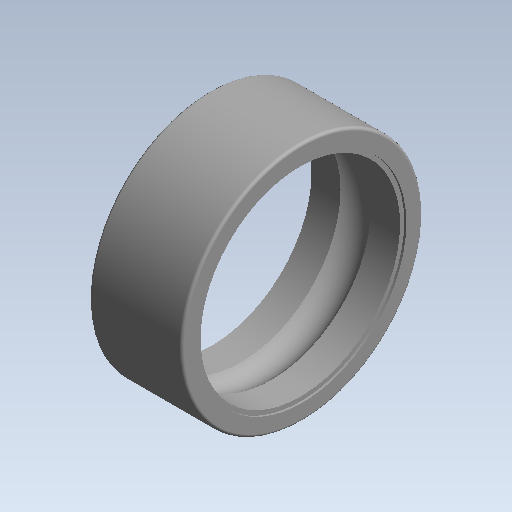
# Autodesk Inventor part: W686ZZ Outer ring
Saved by Autodesk Inventor 2021.3 (Build 253353010, 353A)
## iProperties
Part Number: W686ZZ Outer ring
Material: 一般
Catalog Web Link: www.cadenas.de
Description: Six types or-Metric system sizes
Vendor: NTN
Document SubType Name: Modeling
Designer: partserver
Manufacturer: NTN
Mass: 0.190628 g
Surface Area: 4.63679 cm^2
Volume: 0.190628 cm^3
Density: 1 g/cm^3
Appearance: PSOLRGB-192-192-192
Category: PARTsolutions
Company: NTN
PSOL_IDENT_0: {$CADENAS_DATA\23d-libs\ntn\ball_roller_bearings\miniature_extra_small_bb\metric_system_sizes\mss_or
PSOL_IDENT_1: .prj},183 {VTYP=3D},{NB=W686ZZ Outer ring},{LINA=W686ZZ Outer ring},{NN=Six types or},{DATE=23.10.20
PSOL_IDENT_2: 20 01:13:35},{GEOMDATE=06.03.2020 10:07:12},{VERSION=},{LINEID=12860},{WBVAR=},{WBNUMERIC=}  {NB=W68
PSOL_IDENT_3: 6ZZ Outer ring},{LINA=W686ZZ Outer ring},{KT=DUMMY},{IDNR=},{SD=6.0},{D=13},{B=3.5},{R=0.15},{ORDER=
PSOL_IDENT_4: W686ZZ},{CR=1 080},{COR=440},{CRF=110},{CORF=45},{LSG=39 000},{LSO=46 000},{MASS=1.90},{D1=15.0},{D2=
PSOL_IDENT_5: 15.2},{C1=1.0},{C2=1.1},{ORDER1=686},{WSS=W686ZZ},{WDS=ZZ},{UTWF=FL686},{FORSS=FLW686Z},{FORDS=ZZ},{
PSOL_IDENT_6: DA1=7},{DA2=7,2},{DA=11,8},{RAS=0,15},{MASS1=2.20},{B1=5.0},{VERS=3},{X=3.5},{N=8},{O=29.83},{RB=1.0
PSOL_IDENT_7: 36}
NB: W686ZZ Outer ring
NN: Six types or
NT: Metric system sizes
NBSYN: $ORDER. Outer ring
LINA: W686ZZ Outer ring
CATALOG: NTN Corporation
SD: 6
D: 13
B: 3.5
R: 0.15
CR: 1 080
COR: 440
CRF: 110
CORF: 45
LSG: 39 000
LSO: 46 000
MASS: 1.9
D1: 15
D2: 15.2
C1: 1
C2: 1.1
ORDER1: 686
WSS: W686ZZ
WDS: ZZ
UTWF: FL686
FORSS: FLW686Z
FORDS: ZZ
DA1: 7
DA2: 7,2
DA: 11,8
RAS: 0,15
MASS1: 2.2
B1: 5
VERS: 3
SUPPLIER: NTN
ARTICLENO: W686ZZ Outer ring
BOMINFO: W686ZZ Outer ring
CREATOR: CADENAS GmbH
Title: W686ZZ Outer ring
Author: Cadenas PARTsolutions
Comments: Metric system sizes
Autodesk Inventor part; units mm, degrees
sketch "Sketch_3" plane through (0, 0, 0) normal (0, 0, 1) x (1, 0, 0)
  line L0 (5, 0) -> (0, 0)
  line L1 (0, 5.604) -> (0.1125, 5.604)
  line L2 (0.1125, 5.604) -> (0.1125, 5.38)
  line L3 (0.1125, 5.38) -> (1.6776, 5.38)
  arc A0 (3.3224, 5.38) -> (1.6776, 5.38) centre (2.5, 4.75) ccw
  line L4 (3.3224, 5.38) -> (4.8875, 5.38)
  line L5 (4.8875, 5.38) -> (4.8875, 5.604)
  line L6 (4.8875, 5.604) -> (5, 5.604)
  line L7 (5, 5.604) -> (5, 6.35)
  arc A1 (5, 6.35) -> (4.85, 6.5) centre (4.85, 6.35) ccw
  line L8 (4.85, 6.5) -> (0.15, 6.5)
  arc A2 (0.15, 6.5) -> (0, 6.35) centre (0.15, 6.35) ccw
  line L9 (0, 6.35) -> (0, 5.604)
  constraints: 20 end point, 6 point on circle, 3 centre point
revolve "Revolution1" add sketch "Sketch_3" angle 360 about axis through (5, 0, 0) along (1, 0, 0)
ref_plane "mss_or_XY" through (0, 0, 0) normal (1, 0, 0) x (0, 0, -1)
ref_plane "mss_or_YZ" through (0, 0, 0) normal (0, 0, -1) x (0, 1, 0)
ref_plane "mss_or_ZX" through (0, 0, 0) normal (0, 1, 0) x (1, 0, 0)
ref_plane "mss_or11_XY" through (5, 0, 0) normal (1, 0, 0) x (0, 0, -1)
ref_plane "mss_or11_YZ" through (5, 0, 0) normal (0, 0, -1) x (0, 1, 0)
ref_plane "mss_or11_ZX" through (5, 0, 0) normal (0, 1, 0) x (1, 0, 0)
ref_plane "mss_or2_1_XY" through (1.75, 4.75, 0) normal (1, 0, 0) x (0, 0, -1)
ref_plane "mss_or2_1_YZ" through (1.75, 4.75, 0) normal (0, 0, -1) x (0, 1, 0)
ref_plane "mss_or2_1_ZX" through (1.75, 4.75, 0) normal (0, 1, 0) x (1, 0, 0)
ref_plane "mss_or2_2_XY" through (1.75, 3.3588, 3.3588) normal (1, 0, 0) x (0, 0, -1)
ref_plane "mss_or2_2_YZ" through (1.75, 3.3588, 3.3588) normal (0, 0, -1) x (0, 1, 0)
ref_plane "mss_or2_2_ZX" through (1.75, 3.3588, 3.3588) normal (0, 1, 0) x (1, 0, 0)
ref_plane "mss_or2_3_XY" through (1.75, 0, 4.75) normal (1, 0, 0) x (0, 0, -1)
ref_plane "mss_or2_3_YZ" through (1.75, 0, 4.75) normal (0, 0, -1) x (0, 1, 0)
ref_plane "mss_or2_3_ZX" through (1.75, 0, 4.75) normal (0, 1, 0) x (1, 0, 0)
ref_plane "mss_or2_4_XY" through (1.75, -3.3588, 3.3588) normal (1, 0, 0) x (0, 0, -1)
ref_plane "mss_or2_4_YZ" through (1.75, -3.3588, 3.3588) normal (0, 0, -1) x (0, 1, 0)
ref_plane "mss_or2_4_ZX" through (1.75, -3.3588, 3.3588) normal (0, 1, 0) x (1, 0, 0)
ref_plane "mss_or2_5_XY" through (1.75, -4.75, 0) normal (1, 0, 0) x (0, 0, -1)
ref_plane "mss_or2_5_YZ" through (1.75, -4.75, 0) normal (0, 0, -1) x (0, 1, 0)
ref_plane "mss_or2_5_ZX" through (1.75, -4.75, 0) normal (0, 1, 0) x (1, 0, 0)
ref_plane "mss_or2_6_XY" through (1.75, -3.3588, -3.3588) normal (1, 0, 0) x (0, 0, -1)
ref_plane "mss_or2_6_YZ" through (1.75, -3.3588, -3.3588) normal (0, 0, -1) x (0, 1, 0)
ref_plane "mss_or2_6_ZX" through (1.75, -3.3588, -3.3588) normal (0, 1, 0) x (1, 0, 0)
ref_plane "mss_or2_7_XY" through (1.75, 0, -4.75) normal (1, 0, 0) x (0, 0, -1)
ref_plane "mss_or2_7_YZ" through (1.75, 0, -4.75) normal (0, 0, -1) x (0, 1, 0)
ref_plane "mss_or2_7_ZX" through (1.75, 0, -4.75) normal (0, 1, 0) x (1, 0, 0)
ref_plane "mss_or2_8_XY" through (1.75, 3.3588, -3.3588) normal (1, 0, 0) x (0, 0, -1)
ref_plane "mss_or2_8_YZ" through (1.75, 3.3588, -3.3588) normal (0, 0, -1) x (0, 1, 0)
ref_plane "mss_or2_8_ZX" through (1.75, 3.3588, -3.3588) normal (0, 1, 0) x (1, 0, 0)
ref_plane "mss_or21_1_XY" through (2.5, 4.75, 0) normal (1, 0, 0) x (0, 0, -1)
ref_plane "mss_or21_1_YZ" through (2.5, 4.75, 0) normal (0, 0, -1) x (0, 1, 0)
ref_plane "mss_or21_1_ZX" through (2.5, 4.75, 0) normal (0, 1, 0) x (1, 0, 0)
ref_plane "mss_or21_2_XY" through (2.5, 3.3588, 3.3588) normal (1, 0, 0) x (0, 0, -1)
ref_plane "mss_or21_2_YZ" through (2.5, 3.3588, 3.3588) normal (0, 0, -1) x (0, 1, 0)
ref_plane "mss_or21_2_ZX" through (2.5, 3.3588, 3.3588) normal (0, 1, 0) x (1, 0, 0)
ref_plane "mss_or21_3_XY" through (2.5, 0, 4.75) normal (1, 0, 0) x (0, 0, -1)
ref_plane "mss_or21_3_YZ" through (2.5, 0, 4.75) normal (0, 0, -1) x (0, 1, 0)
ref_plane "mss_or21_3_ZX" through (2.5, 0, 4.75) normal (0, 1, 0) x (1, 0, 0)
ref_plane "mss_or21_4_XY" through (2.5, -3.3588, 3.3588) normal (1, 0, 0) x (0, 0, -1)
ref_plane "mss_or21_4_YZ" through (2.5, -3.3588, 3.3588) normal (0, 0, -1) x (0, 1, 0)
ref_plane "mss_or21_4_ZX" through (2.5, -3.3588, 3.3588) normal (0, 1, 0) x (1, 0, 0)
ref_plane "mss_or21_5_XY" through (2.5, -4.75, 0) normal (1, 0, 0) x (0, 0, -1)
ref_plane "mss_or21_5_YZ" through (2.5, -4.75, 0) normal (0, 0, -1) x (0, 1, 0)
ref_plane "mss_or21_5_ZX" through (2.5, -4.75, 0) normal (0, 1, 0) x (1, 0, 0)
ref_plane "mss_or21_6_XY" through (2.5, -3.3588, -3.3588) normal (1, 0, 0) x (0, 0, -1)
ref_plane "mss_or21_6_YZ" through (2.5, -3.3588, -3.3588) normal (0, 0, -1) x (0, 1, 0)
ref_plane "mss_or21_6_ZX" through (2.5, -3.3588, -3.3588) normal (0, 1, 0) x (1, 0, 0)
ref_plane "mss_or21_7_XY" through (2.5, 0, -4.75) normal (1, 0, 0) x (0, 0, -1)
ref_plane "mss_or21_7_YZ" through (2.5, 0, -4.75) normal (0, 0, -1) x (0, 1, 0)
ref_plane "mss_or21_7_ZX" through (2.5, 0, -4.75) normal (0, 1, 0) x (1, 0, 0)
ref_plane "mss_or21_8_XY" through (2.5, 3.3588, -3.3588) normal (1, 0, 0) x (0, 0, -1)
ref_plane "mss_or21_8_YZ" through (2.5, 3.3588, -3.3588) normal (0, 0, -1) x (0, 1, 0)
ref_plane "mss_or21_8_ZX" through (2.5, 3.3588, -3.3588) normal (0, 1, 0) x (1, 0, 0)
body "Solid1"
